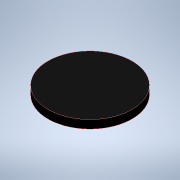
# Autodesk Inventor part: lock1
Saved by Autodesk Inventor 2022 (Build 260153000, 153)
## iProperties
Created: 2021-07-26
Part Number: lock1
Material: Generic
Document SubType Name: Modeling
Designer: Hp
Density: 1 g/cm^3
Appearance: Default
Author: Hp
Autodesk Inventor part; units mm, degrees
ref_plane "YZ Plane" through (0, 0, 0) normal (1, 0, 0) x (0, 1, 0)
ref_plane "XZ Plane" through (0, 0, 0) normal (0, 1, 0) x (-1, 0, 0)
ref_plane "XY Plane" through (0, 0, 0) normal (0, 0, 1) x (1, 0, 0)
sketch "Sketch1" plane through (0, 0, 0) normal (0, 1, 0) x (-1, 0, 0)
  circle A0 centre (10.8306, 18.7601) radius 5.0672
  point P0 (0, 0)
  dimension "d0" = 1
  constraints: 1 centre point
extrude "Extrusion1" add sketch "Sketch1" along normal blind 1
body "Solid1"
